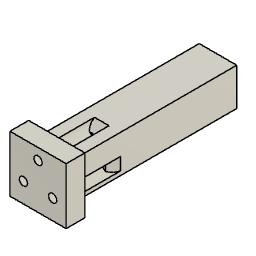
gurigri_square_peg_48mm_y_torgue (Autodesk Fusion 360 design; units mm, degrees)
Autodesk Fusion 360 part; units mm, degrees
box "直方体プリミティブ1" add length 27 width 25 height 5 placed x (0, 1, 0) y (-1, 0, 0) z (0, 0, 1) at (30, 0, 0) makes body 1
sketch "スケッチ2" plane through (0, 0, 5) normal (0, 0, 1) x (-1, 0, 0)
  line L0 (-30, -27) -> (-5, -27)
  line L1 (-5, -27) -> (-5, 0)
  line L2 (-5, 0) -> (-30, 0)
  line L3 (-30, 0) -> (-30, -27)
sketch "スケッチ3" plane through (0, 0, 5) normal (0, 0, 1) x (-1, 0, 0)
  line L0 (0, 0) -> (-35, -40)
  line L1 (-35, -40) -> (-35, 0)
  line L2 (-35, 0) -> (0, -40)
  constraint coincident L0.start origin
  constraint vertical L1
sketch "スケッチ4" plane through (0, 0, 5) normal (0, 0, 1) x (-1, 0, 0)
  line L0 (-17.5, -20) -> (-17.5, 0)
  line L1 (-17.5, 0) -> (-17.5, -5)
  constraint vertical L0
  constraint coincident L0 L1.end
sketch "スケッチ5" plane through (0, 0, 5) normal (0, 0, 1) x (-1, 0, 0)
  line L0 (-17.5, -5) -> (-25, -5)
  line L1 (-25, -5) -> (-10, -5)
  line L2 (-10, -5) -> (-10, 0)
  line L3 (-10, 0) -> (-25, 0)
  line L4 (-25, 0) -> (-25, -5)
  constraint horizontal L0
  constraint parallel L0 L1
  constraint perpendicular L1 L2
  constraint perpendicular L2 L3
  constraint perpendicular L1 L4
box "直方体プリミティブ2" add length 5 width 15 height 15 placed x (0, -1, 0) y (1, 0, 0) z (0, 0, 1) at (10, 5, 5) bodies 1
sketch "スケッチ7" plane through (0, 5, 0) normal (0, 1, 0) x (-1, 0, 0)
  line L0 (-25, 20) -> (-25, 5)
  line L1 (-25, 5) -> (-10, 5)
  line L2 (-10, 5) -> (-10, 20)
  line L3 (-10, 20) -> (-25, 20)
  line L4 (-25, 20) -> (-10, 5)
  line L5 (-10, 20) -> (-25, 5)
  constraint coincident L0.start L3.end
  constraint coincident L1.end L2.start
  constraint coincident L2.end L3.start
  constraint coincident L0.end L1.start
sketch "スケッチ8" plane through (0, 5, 0) normal (0, 1, 0) x (-1, 0, 0)
  circle A0 centre (-17.5, 12.5) radius 4.5
  line L0 (-17.5, 17) -> (-21.3971, 10.25)
  line L1 (-21.3971, 10.25) -> (-13.6029, 10.25)
  line L2 (-13.6029, 10.25) -> (-17.5, 17)
  point P0 (-17.5, 12.5)
  dimension "d11" = 9
  constraint coincident P0 A0.centre
  constraint coincident A0 L0.start
  measures "d11" diameter of A0
hole "穴1" at (13.6029, 5, 10.25) direction (0, -1, 0) diameter 2.2 depth 5 tip angle 180 bodies 1
hole "穴2" at (21.3971, 5, 10.25) direction (0, -1, 0) diameter 2.2 depth 5 tip angle 180 bodies 1
hole "穴3" at (17.5, 5, 17) direction (0, -1, 0) diameter 2.2 depth 5 tip angle 180 bodies 1
sketch "スケッチ12" plane through (0, 0, 5) normal (0, 0, 1) x (-1, 0, 0)
  line L0 (-10, -5, 15) -> (-10, -17, 15)
  line L1 (-10, -17, 15) -> (-25, -17, 15)
  line L2 (-25, -17, 15) -> (-25, -5, 15)
sketch "スケッチ14" plane through (0, 5, 0) normal (0, 1, 0) x (-1, 0, 0)
  line L0 (-17.5, 12.5) -> (-12.5, 12.5)
  dimension "d39" = 5
  constraint horizontal L0
  measures "d39" distance of L0.start L0.end
sketch "スケッチ15" plane through (0, 5, 0) normal (0, 1, 0) x (-1, 0, 0)
  line L0 (-12.5, 12.5) -> (-12.5, 17.5)
  line L1 (-12.5, 17.5) -> (-22.5, 17.5)
  line L2 (-22.5, 17.5) -> (-22.5, 12.5)
  line L3 (-22.5, 12.5) -> (-22.5, 7.5)
  line L4 (-22.5, 7.5) -> (-12.5, 7.5)
  line L5 (-12.5, 7.5) -> (-12.5, 12.5)
  dimension "d40" = 5
  dimension "d41" = 10
  dimension "d42" = 5
  dimension "d43" = 5
  dimension "d44" = 10
  constraint vertical L0
  constraint perpendicular L0 L1
  constraint perpendicular L1 L2
  constraint parallel L2 L3
  constraint perpendicular L3 L4
  measures "d40" distance of L0.start L0.end
  measures "d41" distance of L0.end L1.end
  measures "d42" distance of L1.end L2.end
  measures "d43" distance of L2.end L3.end
  measures "d44" distance of L3.end L4.end
box "直方体プリミティブ6" add length 10 width 10 height 43 placed x (0, 0, -1) y (-1, 0, 0) z (0, 1, 0) at (22.5, 0, 17.5) separate body makes body 2
move_body "移動5" bodies 2 to x (1, 0, 0) y (0, 1, 0) z (0, 0, 1) at (0, 17, 0)
cylinder "円柱プリミティブ2" add diameter 4 height 1 placed x (1, 0, 0) y (0, 0, -1) z (0, 1, 0) at (17.5, 5, 17) separate body makes body 3
sketch "スケッチ18" plane through (0, 5, 0) normal (0, 1, 0) x (-1, 0, 0)
cylinder "円柱プリミティブ3" add diameter 4 height 22 placed x (1, 0, 0) y (0, 0, -1) z (0, 1, 0) at (13.6, 5, 10.25) separate body makes body 4
cylinder "円柱プリミティブ4" add diameter 4 height 10 placed x (1, 0, 0) y (0, 0, -1) z (0, 1, 0) at (21.4, 5, 10.25) separate body makes body 5
move_body "移動6" bodies 5 to x (1, 0, 0) y (0, 1, 0) z (0, 0, 1) at (0, 12, 0)
move_body "移動7" bodies 3 to x (1, 0, 0) y (0, 1, 0) z (0, 0, 1) at (0, 12, 0)
move_face "面をオフセット2" offset 12 1 faces at (17.9301, 17, 16.9352) on bodies 3
move_face "面をオフセット3" offset 12 1 faces at (21.8301, 17, 10.1852) on bodies 5
move_face "面を移動1" by (0, -12, 0) 1 faces at (15.8333, 17, 14.1667) on bodies 2
box "直方体プリミティブ7" cut length 5 width 25 height 30 placed x (0, 0, -1) y (-1, 0, 0) z (0, 1, 0) at (30, 0, 5) bodies 1
combine "結合1" operation add target body 2 tool bodies 1
move_face "面をオフセット4" offset -1 1 faces at (17.9301, 18, 16.9352) on bodies 3
move_face "面をオフセット5" offset -12 1 faces at (13.8307, 27, 9.6562) on bodies 4
move_face "面をオフセット6" offset -12 1 faces at (21.6307, 27, 9.6562) on bodies 5
move_face "面をオフセット7" offset -12 1 faces at (15.8333, 60, 14.1667) on bodies 2
move_face "面をオフセット8" offset -1 1 faces at (17.9301, 17, 16.9352) on bodies 3
move_face "面をオフセット9" offset -1 1 faces at (17.9301, 16, 16.9352) on bodies 3
combine "結合2" operation cut target body 2 tool bodies 3 4 5
chamfer "面取り1" distance 2 angle 45 3 edges at (15.5635, 10, 17.5) (17.5, 15, 17.5) (19.4365, 10, 17.5) on bodies 2
delete_face "面を削除1" 1 faces at (14.4086, 12.3576, 16.8576) on bodies 2
delete_face "面を削除2" 1 faces at (20.5914, 12.3576, 16.8576) on bodies 2
chamfer "面取り2" distance 3 angle 45 2 edges at (12.5, 15, 10.25) (12.5, 10, 11.9203) on bodies 2
delete_face "面を削除3" 1 faces at (13.4649, 12.7018, 13.6577) on bodies 2
delete_face "面を削除4" 1 faces at (16.8385, 16.4879, 16.9879) on bodies 2
chamfer "面取り3" distance 2 angle 45 3 edges at (15.5635, 10, 17.5) (17.5, 15, 17.5) (19.4365, 10, 17.5) on bodies 2
delete_face "面を削除5" 2 faces at (14.4086, 12.3576, 16.8576) (20.5914, 12.3576, 16.8576) on bodies 2
delete_face "面を削除6" 1 faces at (13.7494, 16.7506, 10.909) on bodies 2
chamfer "面取り4" distance 2 angle 45 2 edges at (12.5, 15, 10.25) (12.5, 10, 11.9203) on bodies 2
delete_face "面を削除7" 1 faces at (13.1655, 12.3345, 13.2928) on bodies 2
chamfer "面取り5" distance 2 angle 45 2 edges at (22.5, 15, 10.25) (22.5, 10, 11.9203) on bodies 2
delete_face "面を削除8" 1 faces at (21.8345, 12.3345, 13.2928) on bodies 2
